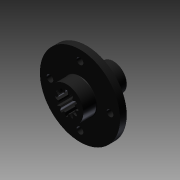
# Autodesk Inventor part: Keyang-12
Saved by Autodesk Inventor 2011 (Build 150239000, 239)
## iProperties
Shininess: 64.0
Length Units: 11272
Angle Units: 11279
Time Units: 11290
Mass Units: 11286
Length Display Precision: 3
Angle Display Precision: 2
Category: Motors
Created: 2007-12-05
Material: ABS Plastic
Document SubType Name: Modeling
Density: 1.06 g/cm^3
Project: FIRST
Description: Coupler for Keyang 12 Tooth Motor
Vendor: Pelham Plastics
Mass: 45.5842 g
Surface Area: 172.303 cm^2
Volume: 43.004 cm^3
Part Number: Keyang-12
Density: 0.0
Volumn: 0.0
Area: 0.0
PropertySet Name: Model Information
Control State: 0
Master: False
Checked Out: False
Title: Coupler, Keyang 12 Tooth Motor
Author: Autodesk, Inc.
Autodesk Inventor part; units mm, degrees
ref_plane "YZ Plane" through (0, 0, 0) normal (1, 0, 0) x (0, 1, 0)
ref_plane "XZ Plane" through (0, 0, 0) normal (0, 1, 0) x (-1, 0, 0)
ref_plane "XY Plane" through (0, 0, 0) normal (0, 0, 1) x (1, 0, 0)
sketch "Sketch1" plane through (0, 0, 0) normal (0, 0, 1) x (1, 0, 0)
  circle A0 centre (0, 0) radius 38.1
  dimension "d2" = 76.2
  constraints: 1 centre point
  measures "d2" diameter of A0
extrude "Extrusion1" add sketch "Sketch1" along normal mid plane 6.35
sketch "Sketch2" plane through (0, 0, 3.175) normal (0, 0, 1) x (1, 0, 0)
  circle A0 centre (0, 0) radius 38.1 projected
  point P0 (0, 28.575)
  dimension "d3" = 0
  dimension "d4" = 28.575
  measures "d3" horizontal distance of A0.centre point (0, 28.575)
  measures "d4" distance of A0.centre point (0, 28.575)
hole "Mounting Hole" at (0, 28.575, 3.175) direction (0, 0, -1) diameter 6.35 end through all
pattern_circular "Circular Pattern1" count 4 over 360 about axis through (0, 0, 0) along (0, 0, 1) of "Mounting Hole"
sketch "Sketch5" plane through (0, 0, -3.175) normal (0, 0, -1) x (-1, 0, 0)
  circle A0 centre (0, 0) radius 38.1 projected
  circle A1 centre (0, 0) radius 14.9225
  dimension "d27" = 29.845
  constraints: 1 centre point, 1 coincident
  measures "d27" diameter of A1
extrude "Extrusion4" add sketch "Sketch5" along normal blind 25.4 draft -5 contours A1
sketch "Sketch6" plane through (0, 0, -28.575) normal (0, 0, -1) x (-1, 0, 0)
  circle A0 centre (0, 0) radius 12.7003 projected
  arc A1 (2.3812, -7.6374) -> (-2.3813, -7.6374) centre (0, 0) ccw
  line L0 (-2.3813, -7.6374) -> (-2.3812, -10.3188)
  line L1 (-2.3812, -10.3188) -> (2.3813, -10.3188)
  line L2 (2.3813, -10.3188) -> (2.3812, -7.6374)
  dimension "d31" = 16
  dimension "d32" = 4.7625
  dimension "d33" = 10.3187
  constraints: 6 end point, 2 parallel, 2 point on circle, 1 centre point, 1 coincident, 1 perpendicular, 1 vertical
  measures "d31" diameter of A1
  measures "d32" distance of L0.end L1.end
  measures "d33" distance from line of L1 A0.centre
extrude "Extrusion5" cut sketch "Sketch6" against normal blind 28.575 contours L2 L1 L0 A1
sketch "Sketch7" plane through (0, 0, 0) normal (0, 0, -1) x (-1, 0, 0)
  arc A0 (2.3812, -7.6374) -> (-2.3813, -7.6374) centre (0, 0) ccw projected
  point P0 (0, 0)
  constraints: 1 coincident
hole "Hole2" at (0, 0, 0) direction (0, 0, 1) diameter 9.525 end through all
sketch "Sketch3" plane through (0, 0, 3.175) normal (0, 0, 1) x (1, 0, 0)
  circle A0 centre (0, 0) radius 38.1 projected
  circle A1 centre (0, 0) radius 15.875
  dimension "d15" = 31.75
  constraints: 1 centre point, 1 coincident
  measures "d15" diameter of A1
extrude "Extrusion2" add sketch "Sketch3" along normal blind 12.7 contours A1
sketch "Sketch8" plane through (0, 0, 15.875) normal (0, 0, 1) x (1, 0, 0)
  circle A0 centre (0, 0) radius 15.875 projected
  constraints: 1 coincident
hole "Hole3" at (0, 0, 15.875) direction (0, 0, -1) diameter 16.2 depth 14.986
sketch "Sketch4" plane through (0, 0, 15.875) normal (0, 0, 1) x (1, 0, 0)
  circle A0 centre (0, 0) radius 15.875 projected
  circle A1 centre (0, 0) radius 8.1 projected
  arc A2 (-6.1113, 9.1462) -> (-4.9718, 5.6692) centre (3.287, 10.3011) ccw
  arc A3 (-4.9718, 5.6692) -> (-5.6692, 4.9718) centre (0, 0) ccw
  arc A4 (-5.6692, 4.9718) -> (-9.1462, 6.1113) centre (-10.3011, -3.287) ccw
  arc A5 (-9.1462, 6.1113) -> (-9.8656, 4.8652) centre (0, 0) ccw
  arc A6 (-9.8656, 4.8652) -> (-7.1403, 2.4238) centre (-2.3039, 10.5645) ccw
  arc A7 (-7.1403, 2.4238) -> (-7.3956, 1.4711) centre (0, 0) ccw
  arc A8 (-7.3956, 1.4711) -> (-10.9764, 0.7194) centre (-7.2775, -7.9972) ccw
  arc A9 (-10.9764, 0.7194) -> (-10.9764, -0.7194) centre (0, 0) ccw
  arc A10 (-10.9764, -0.7194) -> (-7.3956, -1.4711) centre (-7.2775, 7.9972) ccw
  arc A11 (-7.3956, -1.4711) -> (-7.1403, -2.4238) centre (0, 0) ccw
  arc A12 (-7.1403, -2.4238) -> (-9.8656, -4.8652) centre (-2.3039, -10.5645) ccw
  arc A13 (-9.8656, -4.8652) -> (-9.1462, -6.1113) centre (0, 0) ccw
  arc A14 (-9.1462, -6.1113) -> (-5.6692, -4.9718) centre (-10.3011, 3.287) ccw
  arc A15 (-5.6692, -4.9718) -> (-4.9718, -5.6692) centre (0, 0) ccw
  arc A16 (-4.9718, -5.6692) -> (-6.1113, -9.1462) centre (3.287, -10.3011) ccw
  arc A17 (-6.1113, -9.1462) -> (-4.8652, -9.8656) centre (0, 0) ccw
  arc A18 (-4.8652, -9.8656) -> (-2.4238, -7.1403) centre (-10.5645, -2.3039) ccw
  arc A19 (-2.4238, -7.1403) -> (-1.4711, -7.3956) centre (0, 0) ccw
  arc A20 (-1.4711, -7.3956) -> (-0.7194, -10.9764) centre (7.9972, -7.2775) ccw
  arc A21 (-0.7194, -10.9764) -> (0.7194, -10.9764) centre (0, 0) ccw
  arc A22 (0.7194, -10.9764) -> (1.4711, -7.3956) centre (-7.9972, -7.2775) ccw
  arc A23 (1.4711, -7.3956) -> (2.4238, -7.1403) centre (0, 0) ccw
  arc A24 (2.4238, -7.1403) -> (4.8652, -9.8656) centre (10.5645, -2.3039) ccw
  arc A25 (4.8652, -9.8656) -> (6.1113, -9.1462) centre (0, 0) ccw
  arc A26 (6.1113, -9.1462) -> (4.9718, -5.6692) centre (-3.287, -10.3011) ccw
  arc A27 (4.9718, -5.6692) -> (5.6692, -4.9718) centre (0, 0) ccw
  arc A28 (5.6692, -4.9718) -> (9.1462, -6.1113) centre (10.3011, 3.287) ccw
  arc A29 (9.1462, -6.1113) -> (9.8656, -4.8652) centre (0, 0) ccw
  arc A30 (9.8656, -4.8652) -> (7.1403, -2.4238) centre (2.3039, -10.5645) ccw
  arc A31 (7.1403, -2.4238) -> (7.3956, -1.4711) centre (0, 0) ccw
  arc A32 (7.3956, -1.4711) -> (10.9764, -0.7194) centre (7.2775, 7.9972) ccw
  arc A33 (10.9764, -0.7194) -> (10.9764, 0.7194) centre (0, 0) ccw
  arc A34 (10.9764, 0.7194) -> (7.3956, 1.4711) centre (7.2775, -7.9972) ccw
  arc A35 (7.3956, 1.4711) -> (7.1403, 2.4238) centre (0, 0) ccw
  arc A36 (7.1403, 2.4238) -> (9.8656, 4.8652) centre (2.3039, 10.5645) ccw
  arc A37 (9.8656, 4.8652) -> (9.1462, 6.1113) centre (0, 0) ccw
  arc A38 (9.1462, 6.1113) -> (5.6692, 4.9718) centre (10.3011, -3.287) ccw
  arc A39 (5.6692, 4.9718) -> (4.9718, 5.6692) centre (0, 0) ccw
  arc A40 (4.9718, 5.6692) -> (6.1113, 9.1462) centre (-3.287, 10.3011) ccw
  arc A41 (6.1113, 9.1462) -> (4.8652, 9.8656) centre (0, 0) ccw
  arc A42 (4.8652, 9.8656) -> (2.4238, 7.1403) centre (10.5645, 2.3039) ccw
  arc A43 (2.4238, 7.1403) -> (1.4711, 7.3956) centre (0, 0) ccw
  arc A44 (1.4711, 7.3956) -> (0.7194, 10.9764) centre (-7.9972, 7.2775) ccw
  arc A45 (0.7194, 10.9764) -> (-0.7194, 10.9764) centre (0, 0) ccw
  arc A46 (-0.7194, 10.9764) -> (-1.4711, 7.3956) centre (7.9972, 7.2775) ccw
  arc A47 (-1.4711, 7.3956) -> (-2.4238, 7.1403) centre (0, 0) ccw
  arc A48 (-2.4238, 7.1403) -> (-4.8652, 9.8656) centre (-10.5645, 2.3039) ccw
  arc A49 (-4.8652, 9.8656) -> (-6.1113, 9.1462) centre (0, 0) ccw
  constraints: 96 point on circle, 48 centre point, 146 other
extrude "Extrusion3" cut sketch "Sketch4" against normal up to surface (14.986 mm away) contours A1 A32 A31 A30 A28 A27 A26 A24 A23 A22 A20 A19 A18 A16 A15 A14 A12 A11 A10 A8 A7 A6 A4 A3 A2 A48 A47 A46 A44 A43 A42 A40 A39 A38 A36 A35 A34 | A1 A34 A33 A32 | A1 A38 A37 A36 | A30 A29 A28 A1 | A1 A42 A41 A40 | A26 A25 A24 A1 | A1 A46 A45 A44 | A22 A21 A20 A1 | A1 A2 A49 A48 | A18 A17 A16 A1 | A1 A6 A5 A4 | A14 A13 A12 A1 | A1 A10 A9 A8
fillet "Fillet1" radius 0.508 2 edges at (14.9225, 0, -3.175) (-15.875, 0, 3.175)
body "Solid1"
